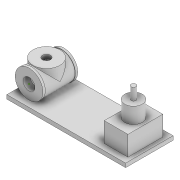
# Autodesk Inventor part: Ventilrohr
Saved by Autodesk Inventor 2021 (Build 250183000, 183)
## iProperties
Created: 2021-06-23
Part Number: Ventilrohr
Material: Generisch
Document SubType Name: Modeling
Designer: stroh
Density: 1 g/cm^3
Appearance: Vorgabe
Author: stroh
Autodesk Inventor part; units mm, degrees
ref_plane "YZ Plane" through (0, 0, 0) normal (1, 0, 0) x (0, 1, 0)
sketch "Skizze7" plane through (0, 0, 0) normal (0, 0, 1) x (1, 0, 0)
  line L0 (-23.8, 0) -> (23.8, 0) projected
  line L1 (0, -23.8) -> (0, 23.8) projected
  circle A0 centre (0, 0) radius 17
  dimension "d18" = 34
  constraints: 1 centre point, 1 coincident
  measures "d18" diameter of A0
extrude "Extrusion7" add sketch "Skizze7" along normal blind 44
sketch "Skizze8" plane through (0, 0, 44) normal (0, 0, 1) x (1, 0, 0)
  circle A0 centre (0, 0) radius 13
  dimension "d21" = 26
  constraints: 1 centre point, 1 coincident
  measures "d21" diameter of A0
extrude "Extrusion8" cut sketch "Skizze8" against normal blind 44
ref_plane "Arbeitsebene2" through (0, 17, 0) normal (0, 1, 0) x (-1, 0, 0)
sketch "Skizze9" plane through (0, 17, 0) normal (0, 1, 0) x (-1, 0, 0)
  circle A0 centre (0, 22) radius 17
  line L0 (17, 44) -> (-17, 44) projected
  point P0 (0, 0)
  dimension "d25" = 34
  dimension "d26" = 22
  constraints: 1 centre point
  measures "d25" diameter of A0
  measures "d26" distance from line of L0 A0.centre
extrude "Extrusion9" add sketch "Skizze9" along normal blind 1 and the other way blind 17
sketch "Skizze10" plane through (0, 0, 44) normal (0, 0, 1) x (1, 0, 0)
  circle A0 centre (0, 0) radius 13
  constraints: 1 centre point, 1 coincident
extrude "Extrusion10" cut sketch "Skizze10" against normal blind 44
sketch "Skizze11" plane through (0, 18, 22) normal (0, 1, 0) x (1, 0, 0)
  circle A0 centre (0, 0) radius 5
  point P0 (0, 22)
  dimension "d33" = 10
  constraints: 1 centre point
  measures "d33" diameter of A0
extrude "Extrusion11" cut sketch "Skizze11" against normal blind 20
sketch "Skizze12" plane through (0, 0, 44) normal (0, 0, 1) x (1, 0, 0)
  point P0 (0, 0)
  point P1 (0, 0)
sketch "Skizze13" plane through (0, 0, 44) normal (0, 0, 1) x (1, 0, 0)
  circle A0 centre (0, 0) radius 7.5
  circle A1 centre (0, 0) radius 13
  dimension "d36" = 15
  constraints: 2 centre point, 2 coincident
  measures "d36" diameter of A0
extrude "Extrusion12" add sketch "Skizze13" against normal blind 44
sketch "Skizze14" plane through (0, 0, 44) normal (0, 0, 1) x (1, 0, 0)
  circle A0 centre (0, 0) radius 13
  dimension "d39" = 26
  constraints: 1 centre point, 1 coincident
  measures "d39" diameter of A0
extrude "Extrusion13" cut sketch "Skizze14" against normal blind 35
sketch "Skizze15" plane through (0, 0, 44) normal (0, 0, 1) x (1, 0, 0)
  circle A0 centre (0, 0) radius 7.5
  circle A1 centre (0, 0) radius 13
  constraints: 2 centre point, 2 coincident
extrude "Extrusion14" add sketch "Skizze15" against normal blind 9
sketch "Skizze16" plane through (0, 0, 44) normal (0, 0, 1) x (1, 0, 0)
  circle A0 centre (0, 0) radius 13 projected
  circle A1 centre (0, 0) radius 17.5
  circle A2 centre (0, 0) radius 17 projected
  circle A3 centre (0, 0) radius 17
  dimension "d44" = 35
  dimension "d45" = 34
  constraints: 2 centre point, 2 coincident
  measures "d44" diameter of A1
  measures "d45" diameter of A3
extrude "Extrusion15" add sketch "Skizze16" against normal blind 3 contours A1
sketch "Skizze17" plane through (0, 0, 0) normal (0, 0, -1) x (-1, 0, 0)
  circle A0 centre (0, 0) radius 17
  circle A1 centre (0, 0) radius 17.5
  dimension "d48" = 35
  dimension "d49" = 34
  constraints: 2 centre point, 2 coincident
  measures "d48" diameter of A1
  measures "d49" diameter of A0
extrude "Extrusion16" add sketch "Skizze17" against normal blind 3
ref_plane "Arbeitsebene4" through (0, -17.5, 0) normal (0, 1, 0) x (-1, 0, 0)
sketch "Skizze21" plane through (0, -17.5, 0) normal (0, 1, 0) x (-1, 0, 0)
  line L0 (20, -8) -> (-130, -8)
  line L1 (-130, -8) -> (-130, 52)
  line L2 (-130, 52) -> (20, 52)
  line L3 (20, 52) -> (20, -8)
  circle A0 centre (0, 22) radius 5 projected
  line L4 (-67, 44) -> (-97, 44) projected
  point P0 (0, 0)
  dimension "d74" = 60
  dimension "d75" = 150
  dimension "d76" = 20
  dimension "d77" = 8
  constraints: 8 end point, 2 parallel, 1 horizontal, 1 perpendicular
  measures "d74" distance between parallel lines of L2 L0
  measures "d75" distance of L0.start L0.end
  measures "d76" distance from line of A0.centre L3
  measures "d77" distance between parallel lines of L4 L2
extrude "Extrusion20" add sketch "Skizze21" against normal blind 5
sketch "Skizze22" plane through (0, -17.5, 0) normal (0, 1, 0) x (1, 0, 0)
  line L0 (95, 0) -> (125, 0)
  line L1 (125, 0) -> (125, -44)
  line L2 (125, -44) -> (95, -44)
  line L3 (95, -44) -> (95, 0)
  line L4 (130, 8) -> (-20, 8) projected
  line L5 (130, -52) -> (130, 8) projected
  line L6 (-20, -52) -> (130, -52) projected
  point P0 (0, 0)
  dimension "d80" = 8
  dimension "d81" = 5
  dimension "d82" = 30
  dimension "d83" = 8
  constraints: 8 end point, 2 parallel, 1 horizontal, 1 perpendicular
  measures "d80" distance between parallel lines of L4 L0
  measures "d81" distance between parallel lines of L5 L1
  measures "d82" distance between parallel lines of L1 L3
  measures "d83" distance between parallel lines of L6 L2
extrude "Extrusion21" add sketch "Skizze22" along normal blind 25
sketch "Skizze23" plane through (0, 7.5, 0) normal (0, 1, 0) x (1, 0, 0)
  circle A0 centre (110, -22) radius 11
  line L0 (95, -44) -> (125, -44) projected
  line L1 (95, 0) -> (95, -44) projected
  point P0 (0, 0)
  dimension "d86" = 22
  dimension "d87" = 22
  dimension "d88" = 15
  constraints: 1 centre point
  measures "d86" diameter of A0
  measures "d87" distance from line of L0 A0.centre
  measures "d88" distance from line of L1 A0.centre
extrude "Extrusion22" add sketch "Skizze23" along normal blind 20
sketch "Skizze24" plane through (110, 27.5, 22) normal (0, 1, 0) x (1, 0, 0)
  circle A0 centre (0, 0) radius 3
  point P0 (-110, 22)
  dimension "d91" = 6
  constraints: 1 centre point
  measures "d91" diameter of A0
extrude "Extrusion23" add sketch "Skizze24" along normal blind 15
